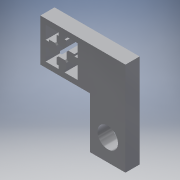
# Autodesk Inventor part: TrackPowerJoint
Saved by Autodesk Inventor 2017 (Build 210142000, 142)
## iProperties
Created: 2005-07-01
Part Number: TrackPowerJoint
Document SubType Name: Modeling
Designer: Administrator
Material: Aluminum-6061
Density: 2.71 g/cm^3
Appearance: Aluminum - Flat
Author: Administrator
Autodesk Inventor part; units mm, degrees
ref_plane "YZ Plane" through (0, 0, 0) normal (1, 0, 0) x (0, 1, 0)
ref_plane "XZ Plane" through (0, 0, 0) normal (0, 1, 0) x (-1, 0, 0)
ref_plane "XY Plane" through (0, 0, 0) normal (0, 0, 1) x (1, 0, 0)
sketch "Sketch1" plane through (0, 0, 0) normal (0, 0, 1) x (1, 0, 0)
  line L0 (-4.1, -22.5) -> (-4.1, -18)
  line L1 (-4.6, -18) -> (-6.8, -18)
  line L2 (-6.8, -18) -> (-6.8, -9.5)
  line L3 (-6.8, -9.5) -> (-4.5, -7.2)
  line L4 (-4.5, -7.2) -> (4.5, -7.2)
  line L5 (4.5, -7.2) -> (6.8, -9.5)
  line L6 (6.8, -9.5) -> (6.8, -18)
  line L7 (4.1, -18) -> (4.1, -22.5)
  line L8 (22.5, -4.1) -> (18, -4.1)
  line L9 (18, -4.6) -> (18, -6.8)
  line L10 (18, -6.8) -> (9.5, -6.8)
  line L11 (9.5, -6.8) -> (7.2, -4.5)
  line L12 (7.2, -4.5) -> (7.2, 4.5)
  line L13 (7.2, 4.5) -> (9.5, 6.8)
  line L14 (9.5, 6.8) -> (18, 6.8)
  line L15 (18, 4.1) -> (22.5, 4.1)
  line L16 (22.5, 22.5) -> (22.5, 4.4)
  line L17 (4.1, 22.5) -> (4.1, 18)
  line L18 (4.6, 18) -> (6.8, 18)
  line L19 (6.8, 18) -> (6.8, 9.5)
  line L20 (6.8, 9.5) -> (4.5, 7.2)
  line L21 (4.5, 7.2) -> (-4.5, 7.2)
  line L22 (-4.5, 7.2) -> (-6.8, 9.5)
  line L23 (-6.8, 9.5) -> (-6.8, 18)
  line L24 (-4.1, 18) -> (-4.1, 22.5)
  line L25 (-22.5, 22.5) -> (-4.4, 22.5)
  line L26 (-22.5, 4.1) -> (-18, 4.1)
  line L27 (-18, 6.8) -> (-9.5, 6.8)
  line L28 (-9.5, 6.8) -> (-7.2, 4.5)
  line L29 (-7.2, 4.5) -> (-7.2, -4.5)
  line L30 (-7.2, -4.5) -> (-9.5, -6.8)
  line L31 (-9.5, -6.8) -> (-18, -6.8)
  line L32 (-18, -6.8) -> (-18, -4.6)
  line L33 (-18, -4.1) -> (-22.5, -4.1)
  line L34 (-22.5, -22.5) -> (-22.5, -4.4)
  line L35 (-4.4, -22.5) -> (-22.5, -22.5)
  line L36 (-6.8, 18) -> (-4.1, 18)
  line L37 (4.1, 18) -> (4.6, 18)
  line L38 (-4.4, 22.5) -> (-3.1, 22.5)
  line L39 (3.1, 22.5) -> (22.5, 22.5)
  line L40 (18, 6.8) -> (18, 4.1)
  line L41 (18, -4.1) -> (18, -4.6)
  line L42 (22.5, 4.4) -> (22.5, 3.1)
  line L43 (22.5, -4.1) -> (22.5, -22.5)
  line L44 (6.8, -18) -> (4.1, -18)
  line L45 (-4.1, -18) -> (-4.6, -18)
  line L46 (22.5, -22.5) -> (4.1, -22.5)
  line L47 (-4.1, -22.5) -> (-4.4, -22.5)
  line L48 (-22.5, -4.4) -> (-22.5, -3.1)
  line L49 (-22.5, 3.1) -> (-22.5, 22.5)
  line L50 (-18, -4.6) -> (-18, -4.1)
  line L51 (-18, 4.1) -> (-18, 6.8)
  line L52 (-24.5, 24.5) -> (24.5, 24.5)
  line L53 (24.5, 24.5) -> (24.5, -24.5)
  line L54 (24.5, -24.5) -> (-24.5, -24.5)
  line L55 (-24.5, -24.5) -> (-24.5, 24.5)
  line L56 (-22.5, 3.1) -> (-17, 3.1)
  line L57 (-17, 5.8) -> (-9.5, 5.8)
  line L58 (-17, 3.1) -> (-17, 5.8)
  line L59 (-8.2, 4.5) -> (-8.2, 0)
  line L60 (-8.2, 4.5) -> (-9.5, 5.8)
  line L61 (-8.2, 4.5) -> (-5.6544, 4.5) construction
  line L62 (-24.5, 0) -> (0, 0)
  line L63 (-22.5, -3.1) -> (-17, -3.1)
  line L64 (-17, -3.1) -> (-17, -5.8)
  line L65 (-17, -5.8) -> (-9.5, -5.8)
  line L66 (-8.2, -4.5) -> (-8.2, 0)
  line L67 (-8.2, -4.5) -> (-9.5, -5.8)
  line L68 (-5.8, -17) -> (-5.8, -9.5)
  line L69 (-4.5, -8.2) -> (-5.8, -9.5)
  line L70 (-4.5, -8.2) -> (0, -8.2)
  line L71 (4.5, -8.2) -> (0, -8.2)
  line L72 (4.5, -8.2) -> (5.8, -9.5)
  line L73 (5.8, -17) -> (5.8, -9.5)
  line L74 (3.1, -17) -> (5.8, -17)
  line L75 (3.1, -22.5) -> (3.1, -17)
  line L76 (-3.1, -17) -> (-5.8, -17)
  line L77 (-3.1, -22.5) -> (-3.1, -17)
  line L78 (17, -5.8) -> (9.5, -5.8)
  line L79 (8.2, -4.5) -> (9.5, -5.8)
  line L80 (8.2, -4.5) -> (8.2, 0)
  line L81 (8.2, 4.5) -> (8.2, 0)
  line L82 (8.2, 4.5) -> (9.5, 5.8)
  line L83 (17, 5.8) -> (9.5, 5.8)
  line L84 (17, 3.1) -> (17, 5.8)
  line L85 (22.5, 3.1) -> (17, 3.1)
  line L86 (17, -3.1) -> (17, -5.8)
  line L87 (22.5, -3.1) -> (17, -3.1)
  line L88 (5.8, 17) -> (5.8, 9.5)
  line L89 (4.5, 8.2) -> (5.8, 9.5)
  line L90 (4.5, 8.2) -> (0, 8.2)
  line L91 (-4.5, 8.2) -> (0, 8.2)
  line L92 (-4.5, 8.2) -> (-5.8, 9.5)
  line L93 (-5.8, 17) -> (-5.8, 9.5)
  line L94 (-3.1, 17) -> (-5.8, 17)
  line L95 (-3.1, 22.5) -> (-3.1, 17)
  line L96 (3.1, 17) -> (5.8, 17)
  line L97 (3.1, 22.5) -> (3.1, 17)
  line L98 (22.5, -4.1) -> (22.5, -3.1)
  line L99 (4.1, -22.5) -> (3.1, -22.5)
  line L100 (-3.1, -22.5) -> (-4.1, -22.5)
  dimension "d7" = 45
  dimension "d8" = 49
  dimension "d9" = 49
  dimension "d11" = 24.5
  dimension "d12" = 24.5
  dimension "d13" = 1
  dimension "d14" = 1
  dimension "d15" = 1
  dimension "d16" = 135
  dimension "d17" = 4.5
  dimension "d20" = 360
  constraints: 202 end point, 23 horizontal, 21 vertical, 6 symmetric about line, 5 point on line, 2 parallel, 1 midpoint, 1 perpendicular, 144 other
  measures "d7" distance between parallel lines of L43 L34
  measures "d8" distance of L53.end L54.end
  measures "d9" distance of L52.end L53.end
  measures "d11" distance from line of L55 L62.end
  measures "d12" distance from line of L62.end L52
  measures "d13" distance between parallel lines of L56 L26
  measures "d14" distance between parallel lines of L51 L58
  measures "d15" distance between parallel lines of L59 L29
  measures "d16" angle of L61 L60
  measures "d17" distance of L59.start L59.end
extrude "Extrusion3" add sketch "Sketch1" along normal blind 20 contours L0 L45 L1 L2 L3 L4 L5 L6 L44 L7 L99 L75 L74 L73 L72 L71 L70 L69 L68 L76 L77 L100 | L48 L63 L64 L65 L67 L66 L62 L29 L30 L31 L32 L50 L33 | L62 L59 L60 L57 L58 L56 L49 L26 L51 L27 L28 L29 | L8 L41 L9 L10 L11 L12 L13 L14 L40 L15 L42 L85 L84 L83 L82 L81 L80 L79 L78 L86 L87 L98 | L38 L95 L94 L93 L92 L91 L90 L89 L88 L96 L97 L39 L17 L37 L18 L19 L20 L21 L22 L23 L36 L24 | L52 L53 L54 L55
sketch "Sketch3" plane through (0, 0, 0) normal (0, 0, -1) x (-1, 0, 0)
  line L0 (24.5, -24.5) -> (24.5, 24.5) projected
  line L1 (24.5, 24.5) -> (-24.5, 24.5) projected
  line L2 (-24.5, 24.5) -> (-24.5, -24.5) projected
  line L3 (-24.5, -24.5) -> (24.5, -24.5) projected
  line L4 (30, 30) -> (-90, 30)
  line L5 (-40, -30) -> (30, -30)
  line L6 (30, -30) -> (30, 30)
  line L7 (-90, -101.9604) -> (-40, -101.9604)
  line L8 (-40, -101.9604) -> (-40, -30)
  line L9 (-90, 30) -> (-90, -101.9604)
  point P0 (0, 0)
  dimension "d25" = 60
  dimension "d26" = 5.5
  dimension "d27" = 49
  dimension "d28" = 5.5
  dimension "d32" = 120
  constraints: 12 end point, 2 vertical, 1 horizontal, 1 parallel
  measures "d25" distance of L5.end L4.start
  measures "d26" distance between parallel lines of L0 L6
  measures "d27" distance of L2.end L0.start
  measures "d28" distance between parallel lines of L4 L1
  measures "d32" distance from line of L6 L4.end
extrude "Extrusion4" add sketch "Sketch3" against normal blind 20
sketch "Sketch4" plane through (0, 0, 20) normal (0, 0, 1) x (1, 0, 0)
  circle A0 centre (65, -71.4443) radius 14.5
  line L0 (40, -101.9604) -> (90, -101.9604) projected
  line L1 (40, -30) -> (40, -101.9604) projected
  point P0 (0, 0)
  dimension "d33" = 29
  dimension "d34" = 50
  dimension "d35" = 25
  constraints: 1 centre point
  measures "d33" diameter of A0
  measures "d34" distance of L0.start L0.end
  measures "d35" distance from line of L1 A0.centre
extrude "Extrusion5" cut sketch "Sketch4" against normal up to next
sketch "Sketch5" plane through (40, -101.9604, 0) normal (0, -1, 0) x (1, 0, 0)
  line L0 (0, 20) -> (50, 20) projected
  line L1 (-70, 20) -> (0, 20) projected
  line L2 (-70, 0) -> (-70, 20) projected
  line L3 (0, 0) -> (-70, 0) projected
  line L4 (50, 0) -> (0, 0) projected
  line L5 (50, 0) -> (50, 20) projected
  circle A0 centre (34, 10) radius 4
  circle A1 centre (18, 10) radius 4
  line L6 (50, 0) -> (0, 0) projected
  line L7 (50, 0) -> (50, 20) projected
  line L8 (0, 20) -> (50, 20) projected
  line L9 (0, 0) -> (0, 20) projected
  point P0 (-40, 0)
  dimension "d38" = 8
  dimension "d39" = 8
  dimension "d40" = 16
  dimension "d41" = 20
  dimension "d42" = 10
  dimension "d43" = 10
  dimension "d44" = 32
  constraints: 2 centre point
  measures "d38" diameter of A0
  measures "d39" diameter of A1
  measures "d40" distance from line of L5 A0.centre
  measures "d41" distance of L4.start L0.end
  measures "d42" distance from line of L4 A0.centre
  measures "d43" distance from line of L4 A1.centre
  measures "d44" distance from line of L5 A1.centre
extrude "Extrusion6" cut sketch "Sketch5" against normal blind 5 contours A0 | A1
equation "\"d9\" = d8"
equation "\"d11\" = 0.5 * d8"
equation "\"d12\" = d11"
equation "\"d26\" = d28"
equation "\"d28\" = -0.5 * d27 + 0.5 * d25"
equation "\"d35\" = 0.5 * d34"
equation "\"d39\" = d38"
equation "\"d42\" = 0.5 * d41"
equation "\"d43\" = d42"
equation "\"d44\" = d40 + 2 * d39"
body "Solid2"
